0.25Offset v5 (Autodesk Fusion 360 design; units mm, degrees)
Autodesk Fusion 360 part; units mm, degrees
sketch "Sketch1" plane through (0, 0, 0) normal (0, 1, 0) x (1, 0, 0)
  circle A0 centre (0, 0) radius 32.5
  circle A1 centre (0, 0) radius 28.5
  dimension "d1" = 65
  dimension "d2" = 57
  constraint coincident A0.centre A1.centre
  measures "d1" diameter of A0
  measures "d2" diameter of A1
extrude "Extrude1" add sketch "Sketch1" along normal blind 10 makes body 1
sketch "Sketch2" plane through (0, 10, 0) normal (0, 1, 0) x (-1, 0, 0)
  circle A0 centre (0, 0) radius 28.5
  circle A1 centre (0, 0) radius 32.5
  circle A2 centre (0, 0) radius 28.5
  circle A3 centre (0, 0) radius 28.25
  circle A4 centre (0, 0) radius 27.25
  dimension "d5" = -0.25
  dimension "d8" = -1.25
extrude "Extrude3" add sketch "Sketch2" along normal blind 30 and the other way blind 5 separate body contours A3 makes body 2
sketch "Sketch3" plane through (0, 0, 0) normal (0, -1, 0) x (1, 0, 0)
  circle A0 centre (0, 0) radius 28.5
  circle A1 centre (0, 0) radius 32.5
  circle A2 centre (0, 0) radius 28.5
  circle A3 centre (0, 0) radius 28.25
extrude "Extrude4" add sketch "Sketch3" against normal blind 10 contours A0 A2 bodies 1 2
fillet "Fillet1" radius 1 1 edges at (26.3382, 5, 10.2156) on bodies 1
chamfer "Chamfer1" distance 0.5 angle 45 1 edges at (26.3382, 40, -10.2156) on bodies 1 2
ref_plane "WorkPlane1" through (28.25, 26.044, 0) normal (1, 0, 0) x (0, 0, 1)
sketch "Sketch4" plane through (28.25, 26.044, 0) normal (1, 0, 0) x (0, 0, -1)
  line L0 (28.25, -16.044) -> (-28.25, -16.044)
  line L1 (28.25, 13.456) -> (-28.25, 13.456)
  line L2 (0, 0) -> (9.3571, 0) construction
  line L3 (9.3571, 0) -> (9.3571, 5.9561) construction
  line L4 (9.3571, 5.9561) -> (0, 5.9561) construction
  line L5 (0, 5.9561) -> (0, 0) construction
  dimension "d22" = 10
  text T0 "0.25" font "Arial" height 10 align centre middle in box 9.3571 x 5.9561 at (0, 0) x (1, 0) y (0, 1) spacing 1
  constraint coincident L2.start
emboss "Emboss1" depth -2 profiles "Sketch4" section 1 text T0 onto face at (-28.2149, 29.6667, -1.4081) on bodies 1 bodies 1 makes body 3 at (27.7858, 25.9555, 5.1005)
delete_body "RemoveBody1" bodies 3
equation "d8 = d5 - 1 mm"
